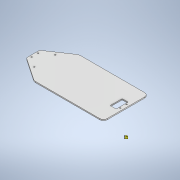
# Autodesk Inventor part: base
Saved by Autodesk Inventor 2020 (Build 240168000, 168)
## iProperties
Created: 2019-08-02
Part Number: base
Material: Generic
Document SubType Name: Modeling
Designer: n10208577
Density: 1 g/cm^3
Appearance: Default
Author: n10208577
Autodesk Inventor part; units mm, degrees
ref_plane "YZ Plane" through (0, 0, 0) normal (1, 0, 0) x (0, 1, 0)
ref_plane "XZ Plane" through (0, 0, 0) normal (0, 1, 0) x (-1, 0, 0)
ref_plane "XY Plane" through (0, 0, 0) normal (0, 0, 1) x (1, 0, 0)
sketch "Sketch1" plane through (0, 0, 0) normal (0, 1, 0) x (-1, 0, 0)
  line L0 (-161.4908, 65.394) -> (-161.4908, 15.394)
  line L1 (19.4074, 75.394) -> (-151.4908, 75.394)
  line L2 (84.8078, 34.3211) -> (27.8032, 72.8242)
  line L3 (-161.4908, 15.394) -> (-161.4908, -34.606)
  circle A0 centre (55.5092, 43.394) radius 1.6
  circle A1 centre (55.5092, -12.606) radius 1.6
  circle A2 centre (82.0092, 24.144) radius 1.6
  circle A3 centre (82.0092, 6.644) radius 1.6
  circle A4 centre (-154.8908, 6.994) radius 1.6
  circle A5 centre (-154.8908, 23.794) radius 1.6
  line L4 (87.0092, 0.6103) -> (87.0092, 30.1777)
  arc A6 (-161.4908, -34.606) -> (-151.4908, -44.606) centre (-151.4908, -34.606) ccw
  arc A7 (-151.4908, 75.394) -> (-161.4908, 65.394) centre (-151.4908, 65.394) ccw
  arc A8 (27.8032, 72.8242) -> (19.4074, 75.394) centre (19.4074, 60.394) ccw
  arc A9 (19.4074, -44.606) -> (27.8032, -42.0362) centre (19.4074, -29.606) ccw
  arc A10 (87.0092, 30.1777) -> (84.8078, 34.3211) centre (82.0092, 30.1777) ccw
  arc A11 (84.8078, -3.5331) -> (87.0092, 0.6103) centre (82.0092, 0.6103) ccw
  line L5 (-151.4908, -44.606) -> (19.4074, -44.606)
  line L6 (27.8032, -42.0362) -> (84.8078, -3.5331)
  line L7 (-151.4908, 15.394) -> (-151.4908, 30.394)
  line L8 (-150.4908, 31.394) -> (-137.4908, 31.394)
  arc A12 (-135.4908, 29.394) -> (-137.4908, 31.394) centre (-137.4908, 29.394) ccw
  arc A13 (-150.4908, 31.394) -> (-151.4908, 30.394) centre (-150.4908, 30.394) ccw
  line L9 (-135.4908, 29.394) -> (-135.4908, 1.394)
  arc A14 (-137.4908, -0.606) -> (-135.4908, 1.394) centre (-137.4908, 1.394) ccw
  line L10 (-137.4908, -0.606) -> (-150.4908, -0.606)
  arc A15 (-151.4908, 0.394) -> (-150.4908, -0.606) centre (-150.4908, 0.394) ccw
  line L11 (-151.4908, 0.394) -> (-151.4908, 15.394)
  point P0 (0, 0)
  constraints: 24 end point, 20 point on circle, 16 centre point
extrude "Extrusion1" add sketch "Sketch1" along normal blind 3
body "Solid1"
